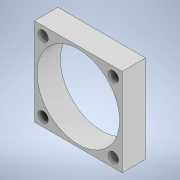
# Autodesk Inventor part: fan
Saved by Autodesk Inventor 2022.1 (Build 261234000, 234)
## iProperties
Created: 2021-08-18
Part Number: fan
Material: Generic
Document SubType Name: Modeling
Designer: robst
Density: 1 g/cm^3
Appearance: Default
Author: robst
Autodesk Inventor part; units mm, degrees
ref_plane "YZ Plane" through (0, 0, 0) normal (1, 0, 0) x (0, 1, 0)
ref_plane "XZ Plane" through (0, 0, 0) normal (0, 1, 0) x (-1, 0, 0)
ref_plane "XY Plane" through (0, 0, 0) normal (0, 0, 1) x (1, 0, 0)
sketch "Sketch1" plane through (0, 0, 0) normal (0, 0, 1) x (1, 0, 0)
  line L0 (-15, -15) -> (15, -15)
  line L1 (15, -15) -> (15, 15)
  line L2 (15, 15) -> (-15, 15)
  line L3 (-15, 15) -> (-15, -15)
  line L4 (-15, -15) -> (15, 15) construction
  line L5 (15, -15) -> (-15, 15) construction
  circle A0 centre (0, 0) radius 14.125
  line L6 (-12, -12) -> (12, -12) construction
  line L7 (12, -12) -> (12, 12) construction
  line L8 (12, 12) -> (-12, 12) construction
  line L9 (-12, 12) -> (-12, -12) construction
  line L10 (-12, -12) -> (12, 12) construction
  line L11 (12, -12) -> (-12, 12) construction
  dimension "d0" = 30
  dimension "d1" = 28.25
  dimension "d2" = 24
  constraints: 24 end point, 5 coincident, 4 midpoint, 4 parallel, 4 perpendicular, 2 horizontal, 1 centre point
  measures "d0" distance of L2.end L0.start
  measures "d1" diameter of A0
  measures "d2" distance of L8.end L6.start
extrude "Extrusion1" add sketch "Sketch1" against normal blind 8
hole "Hole1" at (-12, 12, 0) at (12, 12, 0) at (12, -12, 0) at (-12, -12, 0) direction (0, 0, -1) diameter 3.5 end through all
body "Solid1"
